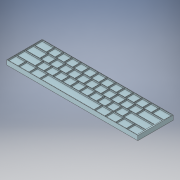
# Autodesk Inventor part: keyboard-base_standard
Saved by Autodesk Inventor 2016 (Build 200138000, 138)
## iProperties
Created: 2016-12-08
Part Number: keyboard-base_standard
Material: Generic
Document SubType Name: Modeling
Designer: Cemra JC
Density: 1 g/cm^3
Appearance: Default
Author: Cemra JC
Autodesk Inventor part; units mm, degrees
ref_plane "YZ Plane" through (0, 0, 0) normal (1, 0, 0) x (0, 1, 0)
ref_plane "XZ Plane" through (0, 0, 0) normal (0, 1, 0) x (-1, 0, 0)
ref_plane "XY Plane" through (0, 0, 0) normal (0, 0, 1) x (1, 0, 0)
sketch "Keyboard Backplane" plane through (0, 0, 0) normal (0, 1, 0) x (-1, 0, 0)
  line L0 (143.25, 38.7) -> (-143.25, 38.7)
  line L1 (-143.25, 38.7) -> (-143.25, -38.7)
  line L2 (-143.25, -38.7) -> (143.25, -38.7)
  line L3 (143.25, -38.7) -> (143.25, 38.7)
  line L4 (143.25, 38.7) -> (-143.25, -38.7) construction
  line L5 (-143.25, 38.7) -> (143.25, -38.7) construction
  point P0 (0, 0)
  point P1 (0, 0)
  dimension "d0" = 77.4
  dimension "d1" = 286.5
  constraints: 12 end point, 2 parallel, 1 coincident, 1 horizontal, 1 midpoint, 1 perpendicular
  measures "d0" distance of L0.end L1.end
  measures "d1" distance of L1.end L2.end
extrude "Keyboard Backplane Body" add sketch "Keyboard Backplane" along normal blind 10
sketch "KeyCap Outlines" plane through (0, 10, 0) normal (0, 1, 0) x (1, 0, 0)
  line L0 (-142.25, 37.7) -> (-115.1, 37.7)
  line L1 (-115.1, 37.7) -> (-115.1, 19.6)
  line L2 (-115.1, 19.6) -> (-142.25, 19.6)
  line L3 (-142.25, 19.6) -> (-142.25, 37.7)
  line L4 (-143.25, -38.7) -> (143.25, -38.7) projected
  line L5 (143.25, -38.7) -> (143.25, 38.7) projected
  line L6 (143.25, 38.7) -> (-143.25, 38.7) projected
  line L7 (-143.25, 38.7) -> (-143.25, -38.7) projected
  line L8 (-114.1, 19.6) -> (-96, 19.6)
  line L9 (-96, 19.6) -> (-96, 37.7)
  line L10 (-96, 37.7) -> (-114.1, 37.7)
  line L11 (-114.1, 37.7) -> (-114.1, 19.6)
  line L12 (-95, 19.6) -> (-76.9, 19.6)
  line L13 (-76.9, 19.6) -> (-76.9, 37.7)
  line L14 (-76.9, 37.7) -> (-95, 37.7)
  line L15 (-95, 37.7) -> (-95, 19.6)
  line L16 (-75.9, 19.6) -> (-57.8, 19.6)
  line L17 (-57.8, 19.6) -> (-57.8, 37.7)
  line L18 (-57.8, 37.7) -> (-75.9, 37.7)
  line L19 (-75.9, 37.7) -> (-75.9, 19.6)
  line L20 (-56.8, 19.6) -> (-38.7, 19.6)
  line L21 (-38.7, 19.6) -> (-38.7, 37.7)
  line L22 (-38.7, 37.7) -> (-56.8, 37.7)
  line L23 (-56.8, 37.7) -> (-56.8, 19.6)
  line L24 (-37.7, 19.6) -> (-19.6, 19.6)
  line L25 (-19.6, 19.6) -> (-19.6, 37.7)
  line L26 (-19.6, 37.7) -> (-37.7, 37.7)
  line L27 (-37.7, 37.7) -> (-37.7, 19.6)
  line L28 (-18.6, 19.6) -> (-0.5, 19.6)
  line L29 (-0.5, 19.6) -> (-0.5, 37.7)
  line L30 (-0.5, 37.7) -> (-18.6, 37.7)
  line L31 (-18.6, 37.7) -> (-18.6, 19.6)
  line L32 (0.5, 19.6) -> (18.6, 19.6)
  line L33 (18.6, 19.6) -> (18.6, 37.7)
  line L34 (18.6, 37.7) -> (0.5, 37.7)
  line L35 (0.5, 37.7) -> (0.5, 19.6)
  line L36 (19.6, 19.6) -> (37.7, 19.6)
  line L37 (37.7, 19.6) -> (37.7, 37.7)
  line L38 (37.7, 37.7) -> (19.6, 37.7)
  line L39 (19.6, 37.7) -> (19.6, 19.6)
  line L40 (38.7, 19.6) -> (56.8, 19.6)
  line L41 (56.8, 19.6) -> (56.8, 37.7)
  line L42 (56.8, 37.7) -> (38.7, 37.7)
  line L43 (38.7, 37.7) -> (38.7, 19.6)
  line L44 (57.8, 19.6) -> (75.9, 19.6)
  line L45 (75.9, 19.6) -> (75.9, 37.7)
  line L46 (75.9, 37.7) -> (57.8, 37.7)
  line L47 (57.8, 37.7) -> (57.8, 19.6)
  line L48 (76.9, 19.6) -> (95, 19.6)
  line L49 (95, 19.6) -> (95, 37.7)
  line L50 (95, 37.7) -> (76.9, 37.7)
  line L51 (76.9, 37.7) -> (76.9, 19.6)
  line L52 (96, 19.6) -> (114.1, 19.6)
  line L53 (114.1, 19.6) -> (114.1, 37.7)
  line L54 (114.1, 37.7) -> (96, 37.7)
  line L55 (96, 37.7) -> (96, 19.6)
  line L56 (115.1, 37.7) -> (142.25, 37.7)
  line L57 (142.25, 37.7) -> (142.25, 19.6)
  line L58 (142.25, 19.6) -> (115.1, 19.6)
  line L59 (115.1, 19.6) -> (115.1, 37.7)
  line L60 (-142.25, 18.6) -> (-110.575, 18.6)
  line L61 (-110.575, 18.6) -> (-110.575, 0.5)
  line L62 (-110.575, 0.5) -> (-142.25, 0.5)
  line L63 (-142.25, 0.5) -> (-142.25, 18.6)
  line L64 (-109.575, 0.5) -> (-91.475, 0.5)
  line L65 (-91.475, 0.5) -> (-91.475, 18.6)
  line L66 (-91.475, 18.6) -> (-109.575, 18.6)
  line L67 (-109.575, 18.6) -> (-109.575, 0.5)
  line L68 (-72.375, 0.5) -> (-72.375, 18.6)
  line L69 (-72.375, 18.6) -> (-90.475, 18.6)
  line L70 (-90.475, 18.6) -> (-90.475, 0.5)
  line L71 (-90.475, 0.5) -> (-72.375, 0.5)
  line L72 (-53.275, 0.5) -> (-53.275, 18.6)
  line L73 (-53.275, 18.6) -> (-71.375, 18.6)
  line L74 (-71.375, 18.6) -> (-71.375, 0.5)
  line L75 (-71.375, 0.5) -> (-53.275, 0.5)
  line L76 (-34.175, 0.5) -> (-34.175, 18.6)
  line L77 (-34.175, 18.6) -> (-52.275, 18.6)
  line L78 (-52.275, 18.6) -> (-52.275, 0.5)
  line L79 (-52.275, 0.5) -> (-34.175, 0.5)
  line L80 (-15.075, 0.5) -> (-15.075, 18.6)
  line L81 (-15.075, 18.6) -> (-33.175, 18.6)
  line L82 (-33.175, 18.6) -> (-33.175, 0.5)
  line L83 (-33.175, 0.5) -> (-15.075, 0.5)
  line L84 (4.025, 0.5) -> (4.025, 18.6)
  line L85 (4.025, 18.6) -> (-14.075, 18.6)
  line L86 (-14.075, 18.6) -> (-14.075, 0.5)
  line L87 (-14.075, 0.5) -> (4.025, 0.5)
  line L88 (23.125, 0.5) -> (23.125, 18.6)
  line L89 (23.125, 18.6) -> (5.025, 18.6)
  line L90 (5.025, 18.6) -> (5.025, 0.5)
  line L91 (5.025, 0.5) -> (23.125, 0.5)
  line L92 (42.225, 0.5) -> (42.225, 18.6)
  line L93 (42.225, 18.6) -> (24.125, 18.6)
  line L94 (24.125, 18.6) -> (24.125, 0.5)
  line L95 (24.125, 0.5) -> (42.225, 0.5)
  line L96 (61.325, 0.5) -> (61.325, 18.6)
  line L97 (61.325, 18.6) -> (43.225, 18.6)
  line L98 (43.225, 18.6) -> (43.225, 0.5)
  line L99 (43.225, 0.5) -> (61.325, 0.5)
  line L100 (80.425, 0.5) -> (80.425, 18.6)
  line L101 (80.425, 18.6) -> (62.325, 18.6)
  line L102 (62.325, 18.6) -> (62.325, 0.5)
  line L103 (62.325, 0.5) -> (80.425, 0.5)
  line L104 (99.525, 0.5) -> (99.525, 18.6)
  line L105 (99.525, 18.6) -> (81.425, 18.6)
  line L106 (81.425, 18.6) -> (81.425, 0.5)
  line L107 (81.425, 0.5) -> (99.525, 0.5)
  line L108 (100.525, 18.6) -> (141.25, 18.6)
  line L109 (141.25, 18.6) -> (141.25, 0.5)
  line L110 (141.25, 0.5) -> (100.525, 0.5)
  line L111 (100.525, 0.5) -> (100.525, 18.6)
  line L112 (-142.25, -0.5) -> (-101.525, -0.5)
  line L113 (-101.525, -0.5) -> (-101.525, -18.6)
  line L114 (-101.525, -18.6) -> (-142.25, -18.6)
  line L115 (-142.25, -18.6) -> (-142.25, -0.5)
  line L116 (-100.525, -0.5) -> (-82.425, -0.5)
  line L117 (-82.425, -0.5) -> (-82.425, -18.6)
  line L118 (-82.425, -18.6) -> (-100.525, -18.6)
  line L119 (-100.525, -18.6) -> (-100.525, -0.5)
  line L120 (-63.325, -18.6) -> (-81.425, -18.6)
  line L121 (-63.325, -0.5) -> (-63.325, -18.6)
  line L122 (-81.425, -18.6) -> (-81.425, -0.5)
  line L123 (-81.425, -0.5) -> (-63.325, -0.5)
  line L124 (-44.225, -18.6) -> (-62.325, -18.6)
  line L125 (-44.225, -0.5) -> (-44.225, -18.6)
  line L126 (-62.325, -18.6) -> (-62.325, -0.5)
  line L127 (-62.325, -0.5) -> (-44.225, -0.5)
  line L128 (-25.125, -18.6) -> (-43.225, -18.6)
  line L129 (-25.125, -0.5) -> (-25.125, -18.6)
  line L130 (-43.225, -18.6) -> (-43.225, -0.5)
  line L131 (-43.225, -0.5) -> (-25.125, -0.5)
  line L132 (-6.025, -18.6) -> (-24.125, -18.6)
  line L133 (-6.025, -0.5) -> (-6.025, -18.6)
  line L134 (-24.125, -18.6) -> (-24.125, -0.5)
  line L135 (-24.125, -0.5) -> (-6.025, -0.5)
  line L136 (13.075, -18.6) -> (-5.025, -18.6)
  line L137 (13.075, -0.5) -> (13.075, -18.6)
  line L138 (-5.025, -18.6) -> (-5.025, -0.5)
  line L139 (-5.025, -0.5) -> (13.075, -0.5)
  line L140 (32.175, -18.6) -> (14.075, -18.6)
  line L141 (32.175, -0.5) -> (32.175, -18.6)
  line L142 (14.075, -18.6) -> (14.075, -0.5)
  line L143 (14.075, -0.5) -> (32.175, -0.5)
  line L144 (51.275, -18.6) -> (33.175, -18.6)
  line L145 (51.275, -0.5) -> (51.275, -18.6)
  line L146 (33.175, -18.6) -> (33.175, -0.5)
  line L147 (33.175, -0.5) -> (51.275, -0.5)
  line L148 (70.375, -18.6) -> (52.275, -18.6)
  line L149 (70.375, -0.5) -> (70.375, -18.6)
  line L150 (52.275, -18.6) -> (52.275, -0.5)
  line L151 (52.275, -0.5) -> (70.375, -0.5)
  line L152 (89.475, -18.6) -> (71.375, -18.6)
  line L153 (89.475, -0.5) -> (89.475, -18.6)
  line L154 (71.375, -18.6) -> (71.375, -0.5)
  line L155 (71.375, -0.5) -> (89.475, -0.5)
  line L156 (90.475, -18.6) -> (140.25, -18.6)
  line L157 (140.25, -18.6) -> (140.25, -0.5)
  line L158 (140.25, -0.5) -> (90.475, -0.5)
  line L159 (90.475, -0.5) -> (90.475, -18.6)
  line L160 (-142.25, -37.7) -> (-119.625, -37.7)
  line L161 (-119.625, -37.7) -> (-119.625, -19.6)
  line L162 (-119.625, -19.6) -> (-142.25, -19.6)
  line L163 (-142.25, -19.6) -> (-142.25, -37.7)
  line L164 (-142.25, -37.7) -> (-119.625, -19.6) construction
  line L165 (-119.625, -37.7) -> (-142.25, -19.6) construction
  line L166 (-96, -37.7) -> (-96, -19.6)
  line L167 (-96, -19.6) -> (-118.625, -19.6)
  line L168 (-118.625, -19.6) -> (-118.625, -37.7)
  line L169 (-118.625, -37.7) -> (-96, -37.7)
  line L170 (-72.375, -37.7) -> (-72.375, -19.6)
  line L171 (-72.375, -19.6) -> (-95, -19.6)
  line L172 (-95, -19.6) -> (-95, -37.7)
  line L173 (-95, -37.7) -> (-72.375, -37.7)
  line L174 (-71.375, -19.6) -> (46.275, -19.6)
  line L175 (46.275, -19.6) -> (46.275, -37.7)
  line L176 (46.275, -37.7) -> (-71.375, -37.7)
  line L177 (-71.375, -37.7) -> (-71.375, -19.6)
  line L178 (47.275, -19.6) -> (69.9, -19.6)
  line L179 (69.9, -19.6) -> (69.9, -37.7)
  line L180 (69.9, -37.7) -> (47.275, -37.7)
  line L181 (47.275, -37.7) -> (47.275, -19.6)
  line L182 (93.525, -37.7) -> (70.9, -37.7)
  line L183 (70.9, -37.7) -> (70.9, -19.6)
  line L184 (70.9, -19.6) -> (93.525, -19.6)
  line L185 (93.525, -19.6) -> (93.525, -37.7)
  line L186 (117.15, -37.7) -> (94.525, -37.7)
  line L187 (94.525, -37.7) -> (94.525, -19.6)
  line L188 (94.525, -19.6) -> (117.15, -19.6)
  line L189 (117.15, -19.6) -> (117.15, -37.7)
  line L190 (140.775, -37.7) -> (118.15, -37.7)
  line L191 (118.15, -37.7) -> (118.15, -19.6)
  line L192 (118.15, -19.6) -> (140.775, -19.6)
  line L193 (140.775, -19.6) -> (140.775, -37.7)
  point P0 (0, 0)
  point P1 (-130.9375, -28.65)
  dimension "d4" = 27.15
  dimension "d5" = 18.1
  dimension "d6" = 1
  dimension "d7" = 1
  dimension "d8" = 18.1
  dimension "d9" = 18.1
  dimension "d10" = 1
  dimension "d11" = 1
  dimension "d14" = 19.1
  dimension "d19" = 27.15
  dimension "d20" = 18.1
  dimension "d21" = 1
  dimension "d22" = 1
  dimension "d23" = 18.1
  dimension "d24" = 31.675
  dimension "d25" = 1
  dimension "d26" = 1
  dimension "d27" = 18.1
  dimension "d28" = 18.1
  dimension "d29" = 1
  dimension "d30" = 1
  dimension "d33" = 19.1
  dimension "d38" = 18.1
  dimension "d39" = 40.725
  dimension "d40" = 1
  dimension "d41" = 1
  dimension "d42" = 18.1
  dimension "d43" = 40.725
  dimension "d44" = 1
  dimension "d45" = 1
  dimension "d46" = 18.1
  dimension "d47" = 18.1
  dimension "d48" = 1
  dimension "d49" = 1
  dimension "d52" = 19.1
  dimension "d57" = 18.1
  dimension "d58" = 49.775
  dimension "d59" = 1
  dimension "d60" = 1
  dimension "d63" = 22.625
  dimension "d64" = 18.1
  dimension "d65" = 1
  dimension "d66" = 1
  dimension "d69" = 23.625
  dimension "d74" = 117.65
  dimension "d75" = 18.1
  dimension "d76" = 1
  dimension "d77" = 1
  dimension "d78" = 22.625
  dimension "d79" = 18.1
  dimension "d80" = 1
  dimension "d81" = 1
  dimension "d84" = 23.625
  constraints: 380 end point, 24 parallel, 17 horizontal, 12 perpendicular, 5 collinear, 2 midpoint, 275 other
  measures "d4" distance of L1.end L2.end
  measures "d5" distance of L0.end L1.end
  measures "d6" distance between parallel lines of L6 L0
  measures "d7" distance between parallel lines of L7 L3
  measures "d8" distance of L10.end L9.end
  measures "d9" distance of L9.end L8.end
  measures "d10" distance between parallel lines of L6 L10
  measures "d11" distance between parallel lines of L1 L11
  measures "d14" distance of L8.start L12.start
  measures "d19" distance of L57.end L58.end
  measures "d20" distance of L56.end L57.end
  measures "d21" distance between parallel lines of L6 L56
  measures "d22" distance between parallel lines of L53 L59
  measures "d23" distance of L60.end L61.end
  measures "d24" distance of L61.end L62.end
  measures "d25" distance between parallel lines of L2 L60
  measures "d26" distance between parallel lines of L7 L63
  measures "d27" distance of L65.end L66.end
  measures "d28" distance of L64.end L65.end
  measures "d29" distance between parallel lines of L8 L66
  measures "d30" distance between parallel lines of L61 L67
  measures "d33" distance of L64.end L68.start
  measures "d38" distance of L108.end L109.end
  measures "d39" distance of L109.end L110.end
  measures "d40" distance between parallel lines of L104 L111
  measures "d41" distance between parallel lines of L58 L108
  measures "d42" distance of L112.end L113.end
  measures "d43" distance of L113.end L114.end
  measures "d44" distance between parallel lines of L7 L115
  measures "d45" distance between parallel lines of L62 L112
  measures "d46" distance of L116.end L117.end
  measures "d47" distance of L117.end L118.end
  measures "d48" distance between parallel lines of L113 L119
  measures "d49" distance between parallel lines of L64 L116
  measures "d52" distance of L117.end L120.start
  measures "d57" distance of L156.end L157.end
  measures "d58" distance of L156.start L156.end
  measures "d59" distance between parallel lines of L153 L159
  measures "d60" distance between parallel lines of L110 L158
  measures "d63" distance of L162.end L161.end
  measures "d64" distance of L161.end L160.end
  measures "d65" distance between parallel lines of L114 L162
  measures "d66" distance between parallel lines of L7 L163
  measures "d69" distance of L160.end L166.start
  measures "d74" distance of L175.end L176.end
  measures "d75" distance of L174.end L175.end
  measures "d76" distance between parallel lines of L170 L177
  measures "d77" distance between parallel lines of L120 L174
  measures "d78" distance of L179.end L180.end
  measures "d79" distance of L178.end L179.end
  measures "d80" distance between parallel lines of L144 L178
  measures "d81" distance between parallel lines of L175 L181
  measures "d84" distance of L179.end L182.start
extrude "Keycap Holes" cut sketch "KeyCap Outlines" against normal blind 3 contours L0 L1 L2 L3 | L11 L10 L9 L8 | L15 L14 L13 L12 | L19 L18 L17 L16 | L23 L22 L21 L20 | L27 L26 L25 L24 | L31 L30 L29 L28 | L35 L34 L33 L32 | L39 L38 L37 L36 | L43 L42 L41 L40 | L47 L46 L45 L44 | L51 L50 L49 L48 | L55 L54 L53 L52 | L56 L57 L58 L59 | L60 L61 L62 L63 | L67 L66 L65 L64 | L71 L70 L69 L68 | L75 L74 L73 L72 | L79 L78 L77 L76 | L83 L82 L81 L80 | L87 L86 L85 L84 | L91 L90 L89 L88 | L95 L94 L93 L92 | L99 L98 L97 L96 | L103 L102 L101 L100 | L107 L106 L105 L104 | L108 L109 L110 L111 | L112 L113 L114 L115 | L116 L117 L118 L119 | L120 L122 L123 L121 | L124 L126 L127 L125 | L128 L130 L131 L129 | L132 L134 L135 L133 | L136 L138 L139 L137 | L140 L142 L143 L141 | L144 L146 L147 L145 | L148 L150 L151 L149 | L152 L154 L155 L153 | L159 L158 L157 L156 | L163 L162 L161 L160 | L169 L168 L167 L166 | L173 L172 L171 L170 | L174 L175 L176 L177 | L178 L179 L180 L181 | L182 L183 L184 L185 | L186 L187 L188 L189 | L190 L191 L192 L193
equation "\"d0\" = b_height"
equation "\"d1\" = b_width"
equation "\"d4\" = b_tab"
equation "\"d5\" = k_width"
equation "\"d6\" = d7"
equation "\"d7\" = b_pad"
equation "\"d8\" = d5"
equation "\"d9\" = d5"
equation "\"d10\" = d6"
equation "\"d11\" = d7"
equation "\"d14\" = d8 + b_pad"
equation "\"d19\" = d4"
equation "\"d20\" = d5"
equation "\"d21\" = d7"
equation "\"d22\" = d7"
equation "\"d23\" = d5"
equation "\"d24\" = b_caps"
equation "\"d25\" = d7"
equation "\"d26\" = d7"
equation "\"d27\" = d5"
equation "\"d28\" = d5"
equation "\"d29\" = b_pad"
equation "\"d30\" = d29"
equation "\"d33\" = d27 + d7"
equation "\"d38\" = d5"
equation "\"d39\" = b_lshift"
equation "\"d40\" = d7"
equation "\"d41\" = d7"
equation "\"d42\" = d5"
equation "\"d43\" = d39"
equation "\"d44\" = d7"
equation "\"d45\" = d7"
equation "\"d46\" = d5"
equation "\"d47\" = d5"
equation "\"d48\" = d7"
equation "\"d49\" = d7"
equation "\"d52\" = d47 + d48"
equation "\"d57\" = d5"
equation "\"d58\" = b_rshift"
equation "\"d59\" = d7"
equation "\"d60\" = d7"
equation "\"d63\" = b_ctrl"
equation "\"d64\" = d5"
equation "\"d65\" = d7"
equation "\"d66\" = d7"
equation "\"d69\" = b_ctrl + b_pad"
equation "\"d74\" = b_space"
equation "\"d75\" = d5"
equation "\"d76\" = d7"
equation "\"d77\" = d7"
equation "\"d78\" = b_ctrl"
equation "\"d79\" = k_width"
equation "\"d80\" = d7"
equation "\"d81\" = d7"
equation "\"d84\" = b_ctrl + b_pad"
equation "\"k_width\" = 18.1"
equation "\"k_height\" = 15"
equation "\"k_taper1\" = 1.5"
equation "\"k_taper2\" = 0.5"
equation "\"k_radius\" = 6"
equation "\"k_wthick\" = 1.5"
equation "\"k_ribthick\" = 1.5"
equation "\"k_ribheight\" = 5"
equation "\"k_poleoff\" = 2.2625"
equation "\"k_poledia\" = 5.54"
equation "\"k_cmxw\" = 1.35"
equation "\"k_cmxl\" = 4.4"
equation "\"s_bwidth\" = 15.6"
equation "\"s_poleh\" = 3.6"
equation "\"s_polebw\" = 5.5"
equation "\"s_polebl\" = 7"
equation "\"b_pad\" = 1"
equation "\"b_tab\" = 27.15"
equation "\"b_caps\" = 31.675"
equation "\"b_lshift\" = 40.725"
equation "\"b_rshift\" = 49.775"
equation "\"b_ctrl\" = 22.625"
equation "\"b_space\" = 117.65"
equation "\"b_width\" = 286.5"
equation "\"b_height\" = 77.4"
equation "\"k_staper\" = 1"
equation "\"k_ltaper\" = 1.5"
equation "\"k_lradius\" = 6"
equation "\"k_sradius\" = 4"
body "Solid1"
